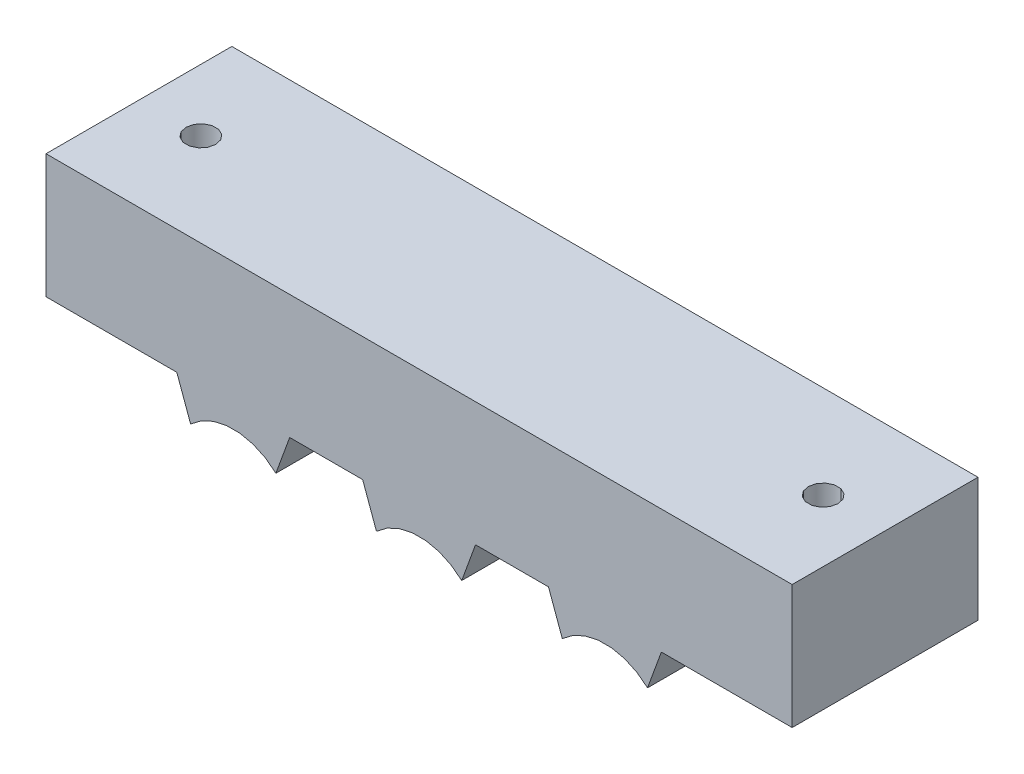
# Autodesk Inventor part: Wire Clamp
Saved by Autodesk Inventor 2014 SP1 (Build 180222100, 222)
## iProperties
Created: 2015-04-18
Part Number: Wire Clamp
Material: Generic
Document SubType Name: Modeling
Designer: tom
Density: 1 g/cm^3
Appearance: Default
Author: tom
Autodesk Inventor part; units mm, degrees
ref_plane "YZ Plane" through (0, 0, 0) normal (1, 0, 0) x (0, 1, 0)
ref_plane "XZ Plane" through (0, 0, 0) normal (0, 1, 0) x (-1, 0, 0)
ref_plane "XY Plane" through (0, 0, 0) normal (0, 0, 1) x (1, 0, 0)
ref_plane "Work Plane1" through (0, 0, 0) normal (0, 0, 1) x (1, 0, 0)
sketch "Sketch1" plane through (0, 0, 0) normal (0, 0, 1) x (1, 0, 0)
  arc A0 (-2.3812, 1.5627) -> (2.3812, 1.5627) centre (0, 1.5627) ccw projected
  line L0 (-2.3812, 1.5627) -> (-3.248, 3.9439) projected
  line L1 (-3.248, 3.9439) -> (-6.277, 3.9439) projected
  line L2 (-6.277, 3.9439) -> (-7.1438, 1.5627) projected
  arc A1 (-11.9063, 1.5627) -> (-7.1438, 1.5627) centre (-9.525, 1.5627) ccw projected
  line L3 (-11.9063, 1.5627) -> (-12.773, 3.9439) projected
  line L4 (-12.773, 3.9439) -> (-19.123, 3.9439) projected
  line L5 (-19.123, 3.9439) -> (-19.123, -1.6123) projected
  line L6 (19.123, -1.6123) -> (-19.123, -1.6123) projected
  line L7 (19.123, -1.6123) -> (19.123, 3.9439) projected
  line L8 (19.123, 3.9439) -> (12.773, 3.9439) projected
  line L9 (12.773, 3.9439) -> (11.9063, 1.5627) projected
  arc A2 (7.1438, 1.5627) -> (11.9063, 1.5627) centre (9.525, 1.5627) ccw projected
  line L10 (7.1438, 1.5627) -> (6.277, 3.9439) projected
  line L11 (6.277, 3.9439) -> (3.248, 3.9439) projected
  line L12 (3.248, 3.9439) -> (2.3812, 1.5627) projected
  line L13 (-12.4172, 4.4519) -> (-11.7101, 2.5091)
  line L14 (-7.3399, 2.5091) -> (-6.6328, 4.4519)
  line L15 (-6.6328, 4.4519) -> (-2.8922, 4.4519)
  line L16 (-2.8922, 4.4519) -> (-2.1851, 2.5091)
  line L17 (2.1851, 2.5091) -> (2.8922, 4.4519)
  line L18 (2.8922, 4.4519) -> (6.6328, 4.4519)
  line L19 (6.6328, 4.4519) -> (7.3399, 2.5091)
  line L20 (11.7101, 2.5091) -> (12.4172, 4.4519)
  line L21 (12.4172, 4.4519) -> (19.123, 4.4519)
  line L22 (-19.123, 4.4519) -> (-12.4172, 4.4519)
  line L23 (-19.123, 4.4519) -> (-19.123, 10.8019)
  line L24 (-19.123, 10.8019) -> (19.123, 10.8019)
  line L25 (19.123, 10.8019) -> (19.123, 4.4519)
  arc A3 (-7.3399, 2.5091) -> (-11.7101, 2.5091) centre (-9.525, 0.2056) ccw
  arc A4 (2.1851, 2.5091) -> (-2.1851, 2.5091) centre (0, 0.2056) ccw
  arc A5 (11.7101, 2.5091) -> (7.3399, 2.5091) centre (9.525, 0.2056) ccw
  point P0 (0, 0)
  dimension "d0" = 0.508
  dimension "d1" = 6.35
  dimension "d5" = 3.175
  dimension "d6" = 3.175
  dimension "d7" = 3.175
  constraints: 30 end point, 6 point on circle, 3 centre point, 2 perpendicular, 1 parallel
  measures "d0" distance between parallel lines of L4 L22
  measures "d1" distance of L22.start L23.end
  measures "d5" radius of A3
  measures "d6" radius of A4
  measures "d7" radius of A5
extrude "Extrusion1" add sketch "Sketch1" against normal blind 9.525 contours L22 L23 L24 L25 L21 L20 A5 L19 L18 L17 A4 L16 L15 L14 A3 L13
sketch "Sketch2" plane through (-19.123, 10.8019, 0) normal (0, 1, 0) x (1, 0, 0)
  circle A0 centre (3.175, 4.7625) radius 0.762 projected
  circle A1 centre (35.0709, 4.7625) radius 0.762 projected
  point P0 (19.123, 0)
extrude "Extrusion2" cut sketch "Sketch2" against normal blind 9.525
body "Solid1"
